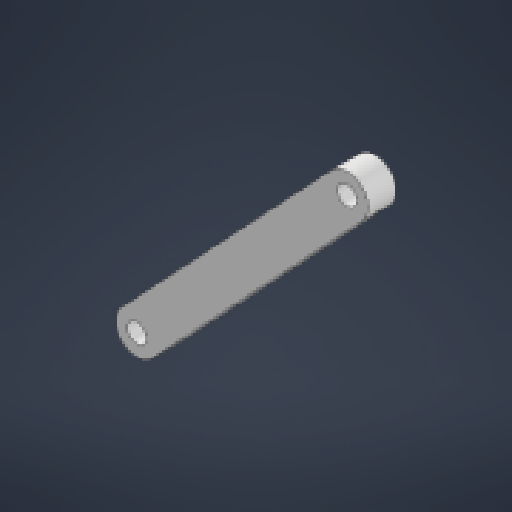
# Autodesk Inventor part: thingy
Saved by Autodesk Inventor 2025.2 (Build 292293000, 293)
## iProperties
Created: 2025-12-05
Part Number: thingy
Material: Generic
Document SubType Name: Modeling
Designer: cloudy
Density: 1 g/cm^3
Appearance: Default
Author: cloudy
Autodesk Inventor part; units mm, degrees
ref_plane "YZ Plane" through (0, 0, 0) normal (1, 0, 0) x (0, 1, 0)
ref_plane "XZ Plane" through (0, 0, 0) normal (0, 1, 0) x (-1, 0, 0)
ref_plane "XY Plane" through (0, 0, 0) normal (0, 0, 1) x (1, 0, 0)
sketch "Sketch1" plane through (0, 0, 0) normal (0, 0, 1) x (1, 0, 0)
  circle A0 centre (38.1, -25.4) radius 2.1844 projected
  circle A1 centre (84.267, 23.8448) radius 2.1844 projected
  circle A2 centre (38.1, -25.4) radius 4.7625
  circle A3 centre (84.267, 23.8448) radius 4.7625
  line L0 (80.7926, 27.1021) -> (31.2119, -25.784)
  line L1 (36.9187, -33.6234) -> (89.3053, 22.2556)
  point P0 (0, 0)
  point P1 (34.6256, -22.1427)
  point P2 (41.5744, -28.6573)
  point P3 (87.7414, 20.5875)
  dimension "d1" = 9.525
  dimension "d0" = 9.525
  constraints: 4 end point, 2 coincident, 2 tangent, 1 centre point, 5 other
  measures "d0" diameter of A2
extrude "Extrusion1" add sketch "Sketch1" along normal blind 6.35
body "Solid1"
